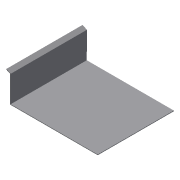
# Autodesk Inventor part: ToteBasin
Saved by Autodesk Inventor 2015 (Build 190159000, 159)
## iProperties
Created: 2015-03-06
Part Number: ToteBasin
Material: Generic
Document SubType Name: Modeling
Designer: Jaden
Density: 1 g/cm^3
Appearance: Default
Author: Jaden
Autodesk Inventor part; units mm, degrees
ref_plane "YZ Plane" through (0, 0, 0) normal (1, 0, 0) x (0, 1, 0)
ref_plane "XZ Plane" through (0, 0, 0) normal (0, 1, 0) x (-1, 0, 0)
ref_plane "XY Plane" through (0, 0, 0) normal (0, 0, 1) x (1, 0, 0)
sketch "Sketch1" plane through (0, 0, 0) normal (0, 0, 1) x (1, 0, 0)
  line L0 (0, 0) -> (-23.2949, 10.1247)
  line L1 (0, 0) -> (25.4, 0) construction
  line L2 (-23.2949, 10.1247) -> (-24.5605, 7.2128)
  line L3 (-24.5605, 7.2128) -> (-4.1774, -1.6463)
  line L4 (-4.1774, -1.6463) -> (173.6226, -1.6463) construction
  line L5 (0, 0) -> (176.276, 0) construction
  line L6 (-4.1774, -1.6463) -> (-4.1774, -141.3463)
  line L7 (-4.1774, -1.6463) -> (135.5226, -1.6463) construction
  line L8 (-4.1774, -141.3463) -> (453.0226, -141.3463)
  line L9 (453.0226, -141.3463) -> (453.0226, -138.1713)
  line L10 (453.0226, -138.1713) -> (-1.0024, -138.1713)
  line L11 (-1.0024, -138.1713) -> (0, 0)
  dimension "d0" = 25.4
  dimension "d1" = 156.509
  dimension "d2" = 3.175
  dimension "d3" = 90
  dimension "d4" = 22.225
  dimension "d5" = 90
  dimension "d22" = 139.7
  dimension "d23" = 90
  dimension "d24" = 457.2
  dimension "d25" = 90
  dimension "d26" = 3.175
  dimension "d27" = 454.025
  dimension "d28" = 90
  constraints: 24 end point, 5 perpendicular, 4 horizontal, 2 equal length, 1 vertical
  measures "d0" distance of L0.start L0.end
  measures "d1" angle of L1 L0
  measures "d2" distance of L0.end L2.end
  measures "d3" angle of L2 L0
  measures "d4" distance of L2.end L3.end
  measures "d5" angle of L3 L2
  measures "d22" distance of L3.end L6.end
  measures "d23" angle of L6 L7
  measures "d24" distance of L6.end L8.end
  measures "d25" angle of L8 L6
  measures "d26" distance of L8.end L9.end
  measures "d27" distance of L9.end L10.end
  measures "d28" angle of L10 L9
extrude "Extrusion3" add sketch "Sketch1" along normal blind 396.875
body "Solid3"
